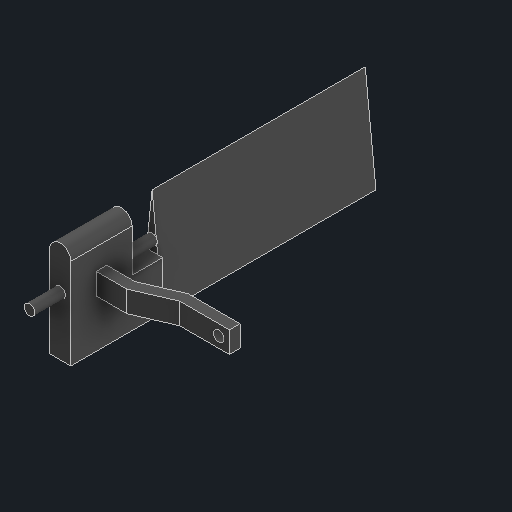
# Autodesk Inventor part: rudder_fin
Saved by Autodesk Inventor 2024 (Build 280153000, 153)
## iProperties
Created: 2022-03-30
Part Number: rudder_fin
Material: Generic
Document SubType Name: Modeling
Designer: kardo
Density: 1 g/cm^3
Appearance: Dark Plastic
Mass: 2.79208 g
Surface Area: 28.6098 cm^2
Volume: 2.79208 cm^3
Author: kardo
Autodesk Inventor part; units mm, degrees
ref_plane "YZ Plane" through (0, 0, 0) normal (1, 0, 0) x (0, 1, 0)
ref_plane "XY Plane" through (0, 0, 0) normal (0, 0, 1) x (1, 0, 0)
derived "parameters_powertrain.ipt"
derived "rudder_base.ipt"
sketch "sk_base" plane through (0, 0, 0) normal (0, 1, 0) x (-1, 0, 0)
  line L0 (16.1, 0) -> (-16.1, 0) construction
  line L1 (0, -4.6) -> (0, 27.6) construction
  line L2 (0, 23) -> (0, 15.5) construction
  line L3 (0, 7.5) -> (0, 0) construction
sketch "sk_length" plane through (0, 0, 0) normal (0, 0, 1) x (1, 0, 0)
  line L0 (0, -62.4) -> (0, 10.4) construction
  line L1 (-6, 0) -> (8, 0) construction
  arc A0 (2, -50) -> (6, -50) centre (4, -50) ccw
  line L2 (2, -50) -> (2, -40)
  line L3 (2, -40) -> (4, -40)
  line L4 (4, -40) -> (4, -2)
  line L5 (4, -2) -> (-4, -2)
  line L6 (-4, -2) -> (-4, 0)
  line L7 (-4, 0) -> (6, 0)
  line L8 (6, 0) -> (6, -50)
  point P0 (0, 0)
  point P1 (0, 10.4)
sketch "sk_joint_base" plane through (0, 0, 0) normal (0, 0, 1) x (1, 0, 0)
  line L0 (2, -40) -> (4, -40) construction
  arc A0 (6, -44) -> (2, -44) centre (4, -44) ccw
  line L1 (2, -44) -> (2, -61)
  line L2 (6, -61) -> (6, -44)
  line L3 (2, -61) -> (6, -61)
  line L4 (2, -50) -> (2, -40) construction
  line L5 (6, 0) -> (6, -50) construction
  arc A1 (2, -50) -> (6, -50) centre (4, -50) ccw construction
  line L6 (4, -40) -> (4, -42) construction
  point P0 (0, 0)
  dimension "d30" = 2
  dimension "d31" = 17
  constraints: 8 end point, 3 point on circle, 2 collinear, 2 perpendicular, 2 tangent, 1 centre point
  measures "d30" distance of L0.end L6.end
  measures "d31" distance from line of L3 A0.centre
sketch "sk_blade_base" plane through (0, 0, 0) normal (0, 0, 1) x (1, 0, 0)
  arc A0 (6, -44) -> (2, -44) centre (4, -44) ccw construction
  line L0 (2, -61) -> (6, -61) projected
  line L1 (2, -61) -> (4, -42)
  line L2 (6, -61) -> (4, -42)
  point P0 (0, 0)
  constraints: 4 end point, 1 point on circle
sketch "sk_axle" plane through (0, 0, 0) normal (0, 0, 1) x (1, 0, 0)
  circle A0 centre (4, -50) radius 1
  point P0 (0, 0)
  dimension "d7" = 2
  constraints: 1 centre point, 1 coincident
  measures "d7" diameter of A0
extrude "extrude_joint" add sketch "sk_joint_base" along normal up to surface (23 mm away)
extrude "extrude_blade" add sketch "sk_blade_base" against normal blind 40
sketch "sk_trim" plane through (0, 0, 0) normal (1, 0, 0) x (0, 1, 0)
  line L0 (-50, 0) -> (-52, 0) projected
  line L1 (-40, 0) -> (-52, 0)
  line L2 (-40, 0) -> (-40, 5.75)
  line L3 (-40, 5.75) -> (-52, 5.75)
  line L4 (-52, 5.75) -> (-52, 0)
  line L5 (-40, 23) -> (-61, 23)
  line L6 (-61, 23) -> (-61, 17.25)
  line L7 (-61, 17.25) -> (-40, 17.25)
  line L8 (-40, 17.25) -> (-40, 23)
  point P0 (0, 0)
  point P1 (0, 23)
  point P2 (-61, 0)
  dimension "d40" = 23
  dimension "d41" = 11.5
  constraints: 16 end point, 4 perpendicular, 3 parallel, 2 collinear, 2 point on line
  measures "d40" distance of point (-40, 0) L5.start
  measures "d41" distance of L2.end L7.end
extrude "trim_joint" cut sketch "sk_trim" along normal through all both and the other way through all
extrude "extrude_axle" add sketch "sk_axle" along normal up to surface (23 mm away)
ref_plane "plane_axle" through (4, -50, 0) normal (0, 1, 0) x (-1, 0, 0)
sketch "sk_arm" plane through (4, -50, 0) normal (0, 1, 0) x (-1, 0, 0)
  line L0 (4, -118.42) -> (4, 46.57) construction
  line L1 (129.6, 0) -> (-49.6, 0) construction
  line L2 (4, -92.5) -> (104, -92.5) construction
  line L3 (104, -92.5) -> (104, 0) construction
  line L4 (0, 12.5) -> (-7.7483, 12.5)
  line L5 (-7.7483, 12.5) -> (-14.6667, 9.5)
  line L6 (-14.6667, 9.5) -> (-22, 9.5)
  line L7 (-24, 9.5) -> (-24, 7.5)
  line L8 (-24, 7.5) -> (-14.2517, 7.5)
  line L9 (-14.2517, 7.5) -> (-7.3333, 10.5)
  line L10 (-7.3333, 10.5) -> (0, 10.5)
  line L11 (-7.3333, 10.5) -> (-14.6667, 10.5) construction
  line L12 (-14.6667, 10.5) -> (-14.6667, 9.5) construction
  line L13 (-22, 9.5) -> (-24, 9.5)
  line L14 (0, 12.5) -> (0, 10.5)
  line L15 (4, 15.5) -> (0, 12.5) construction
  line L16 (0, 10.5) -> (4, 7.5) construction
  point P0 (4, 0)
  point P1 (0, 0)
  dimension "d11" = 100
  dimension "d15" = 102
  dimension "d16" = 126
  dimension "d17" = 2
  dimension "d18" = 2
  dimension "d19" = 2
  dimension "d20" = 2
  dimension "d44" = 100
  constraints: 30 end point, 6 parallel, 4 perpendicular, 3 equal length, 3 point on line, 2 collinear
  measures "d11" distance between parallel lines of L3 L0
  measures "d15" distance from line of L2 L6.end
  measures "d16" distance from line of L6.end L3
  measures "d17" distance between parallel lines of L4 L10
  measures "d18" distance between parallel lines of L6 L8
  measures "d19" distance between parallel lines of L5 L9
  measures "d20" distance of L6.end L7.start
  measures "d44" distance from line of L2 L16.end
extrude "extrude_arm" add sketch "sk_arm" along normal mid plane 4
sketch "sk_rod_drill" plane through (18.6667, -48, 9.5) normal (0, 0, 1) x (1, 0, 0)
  point P0 (-18.6667, 48)
  point P1 (7.3333, -2)
hole "rod_drill" at (26, -50, 9.5) direction (0, 0, -1) diameter 2 end through all
equation "\"d41\" = 0.5 * d40"
equation "\"d15\" = d14 + rudder_rod_joint_up"
equation "\"d16\" = d11 + rudder_rod_joint_right"
equation "\"d14\" = 100"
equation "\"rudder_rod_joint_up\" = 2"
equation "\"rudder_rod_joint_right\" = 26"
body "Solid1"
